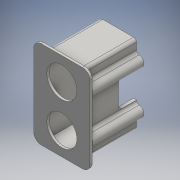
# Autodesk Inventor part: Side Lidar Mount
Saved by Autodesk Inventor 2016 (Build 200138000, 138)
## iProperties
Created: 2017-04-03
Part Number: Side Lidar Mount
Material: Generic
Document SubType Name: Modeling
Designer: BenjaPad
Density: 1 g/cm^3
Appearance: Default
Author: BenjaPad
Autodesk Inventor part; units mm, degrees
ref_plane "YZ Plane" through (0, 0, 0) normal (1, 0, 0) x (0, 1, 0)
ref_plane "XZ Plane" through (0, 0, 0) normal (0, 1, 0) x (-1, 0, 0)
ref_plane "XY Plane" through (0, 0, 0) normal (0, 0, 1) x (1, 0, 0)
sketch "Sketch1" plane through (0, 0, 0) normal (0, 1, 0) x (-1, 0, 0)
  circle A0 centre (0, 13.9) radius 10
  circle A1 centre (0, -13.9) radius 10
  line L0 (-18.75, 29.25) -> (18.75, 29.25)
  line L1 (18.75, 29.25) -> (18.75, -29.25)
  line L2 (18.75, -29.25) -> (-18.75, -29.25)
  line L3 (-18.75, -29.25) -> (-18.75, 29.25)
  line L4 (-18.75, 29.25) -> (18.75, -29.25) construction
  line L5 (18.75, 29.25) -> (-18.75, -29.25) construction
  point P0 (0, 0)
  dimension "d0" = 20
  dimension "d1" = 20
  dimension "d2" = 27.8
  dimension "d3" = 13.9
  dimension "d4" = 37.5
  dimension "d5" = 58.5
  constraints: 12 end point, 2 centre point, 2 midpoint, 2 parallel, 1 horizontal, 1 perpendicular
  measures "d0" diameter of A0
  measures "d1" diameter of A1
  measures "d2" distance of A1.centre A0.centre
  measures "d3" distance of point (0, 0) A1.centre
  measures "d4" distance of L1.end L2.end
  measures "d5" distance of L0.end L1.end
extrude "Extrusion1" add sketch "Sketch1" along normal blind 1.5
sketch "Sketch2" plane through (0, 1.5, 0) normal (0, 1, 0) x (1, 0, 0)
  line L0 (10.25, -24.25) -> (-10.25, -24.25)
  line L1 (-10.25, -24.25) -> (-10.25, 24.25)
  line L2 (-10.25, 24.25) -> (10.25, 24.25)
  line L3 (10.25, 24.25) -> (10.25, -24.25)
  line L4 (10.25, -24.25) -> (-10.25, 24.25) construction
  line L5 (-10.25, -24.25) -> (10.25, 24.25) construction
  line L6 (13.75, -14.5) -> (-13.75, -14.5) construction
  line L7 (-13.75, -14.5) -> (-13.75, 14.5) construction
  line L8 (-13.75, 14.5) -> (13.75, 14.5) construction
  line L9 (13.75, 14.5) -> (13.75, -14.5) construction
  line L10 (13.75, -14.5) -> (-13.75, 14.5) construction
  line L11 (-13.75, -14.5) -> (13.75, 14.5) construction
  circle A0 centre (-13.75, -14.5) radius 1.95
  circle A1 centre (-13.75, 14.5) radius 1.95
  circle A2 centre (13.75, 14.5) radius 1.95
  circle A3 centre (13.75, -14.5) radius 1.95
  arc A4 (12.25, -17.6623) -> (12.25, -11.3377) centre (13.75, -14.5) ccw
  arc A5 (-12.25, 17.6623) -> (-12.25, 11.3377) centre (-13.75, 14.5) ccw
  arc A6 (-12.25, -11.3377) -> (-12.25, -17.6623) centre (-13.75, -14.5) ccw
  line L12 (-12.25, -26.25) -> (12.25, -26.25)
  line L13 (12.25, 26.25) -> (-12.25, 26.25)
  line L14 (-12.25, -17.6623) -> (-12.25, -26.25)
  line L15 (-12.25, -12.9182) -> (-12.25, -14.5)
  line L16 (-12.25, 11.3377) -> (-12.25, -11.3377)
  line L17 (-12.25, 26.25) -> (-12.25, 17.6623)
  line L18 (12.25, 17.6623) -> (12.25, 26.25)
  arc A7 (12.25, 11.3377) -> (12.25, 17.6623) centre (13.75, 14.5) ccw
  line L19 (12.25, -11.3377) -> (12.25, 11.3377)
  line L20 (12.25, -26.25) -> (12.25, -17.6623)
  point P0 (0, 0)
  dimension "d8" = 20.5
  dimension "d9" = 48.5
  dimension "d10" = 27.5
  dimension "d11" = 29
  dimension "d12" = 3.9
  dimension "d13" = 3.9
  dimension "d14" = 3.9
  dimension "d15" = 3.9
  constraints: 42 end point, 17 parallel, 8 centre point, 8 coincident, 8 point on circle, 6 perpendicular, 4 midpoint, 2 horizontal, 2 point on line, 1 tangent
  measures "d8" distance of L1.end L2.end
  measures "d9" distance of L0.end L1.end
  measures "d10" distance of L7.end L8.end
  measures "d11" distance of L6.end L7.end
  measures "d12" diameter of A0
  measures "d13" diameter of A1
  measures "d14" diameter of A2
  measures "d15" diameter of A3
extrude "Extrusion2" add sketch "Sketch2" along normal blind 36
fillet "Fillet1" radius 2 12 edges at (12.25, 19.5, 17.6623) (12.25, 19.5, 11.3377) (12.25, 19.5, -11.3377) (12.25, 19.5, -17.6623) (-12.25, 19.5, -11.3377) (-12.25, 19.5, -17.6623) (-12.25, 19.5, 17.6623) (-12.25, 19.5, 11.3377) (12.25, 19.5, 26.25) (-12.25, 19.5, 26.25) (12.25, 19.5, -26.25) (-12.25, 19.5, -26.25)
fillet "Fillet2" radius 2 24 edges at (12.7729, 1.5, 10.3712) (17.25, 1.5, 14.5) (12.7729, 1.5, 18.6288) (12.25, 1.5, 22.1136) (11.6642, 1.5, 25.6642) (0, 1.5, 26.25) (-11.6642, 1.5, 25.6642) (-12.25, 1.5, 22.1136) (-12.7729, 1.5, 18.6288) (-17.25, 1.5, 14.5) (-12.7729, 1.5, 10.3712) (-12.25, 1.5, 0) (-12.7729, 1.5, -10.3712) (-17.25, 1.5, -14.5) (-12.7729, 1.5, -18.6288) (-12.25, 1.5, -22.1136) (-11.6642, 1.5, -25.6642) (0, 1.5, -26.25) (11.6642, 1.5, -25.6642) (12.25, 1.5, -22.1136) (12.7729, 1.5, -18.6288) (17.25, 1.5, -14.5) (12.7729, 1.5, -10.3712) (12.25, 1.5, 0)
sketch "Sketch3" plane through (12.25, 37.5, 9.0228) normal (1, 0, 0) x (0, 0, -1)
  line L0 (18.0455, -34) -> (0, -34) projected
  line L1 (18.0455, 0) -> (18.0455, -34) projected
  line L2 (0, 0) -> (18.0455, 0) projected
  line L3 (0, -34) -> (0, 0) projected
  line L4 (0.0228, -12) -> (18.0228, -12)
  line L5 (18.0228, -12) -> (18.0228, 12)
  line L6 (18.0228, 12) -> (0.0228, 12)
  line L7 (0.0228, 12) -> (0.0228, -12)
  line L8 (18.0455, 0) -> (0, 0) projected
  line L9 (0.0228, -12) -> (18.0228, 12) construction
  line L10 (18.0228, -12) -> (0.0228, 12) construction
  point P0 (9.0228, -37.5)
  point P1 (9.0228, 0)
  dimension "d21" = 18
  dimension "d22" = 24
  constraints: 12 end point, 3 midpoint, 2 parallel, 1 horizontal, 1 perpendicular
  measures "d21" distance of L6.end L5.end
  measures "d22" distance of L5.end L4.end
extrude "Extrusion3" cut sketch "Sketch3" against normal blind 2 contours L5 L4 L7 L2 | L2 L7 L6 L5
fillet "Fillet3" radius 2 2 edges at (11.25, 25.5, -9) (11.25, 25.5, 9)
fillet "Fillet4" radius 5 4 edges at (18.75, 0.75, -29.25) (-18.75, 0.75, -29.25) (18.75, 0.75, 29.25) (-18.75, 0.75, 29.25)
body "Solid1"
